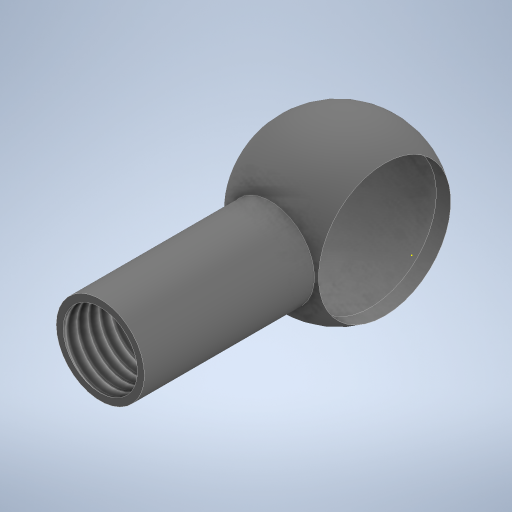
# Autodesk Inventor part: Part1
Saved by Autodesk Inventor 2023 (Build 270158000, 158)
## iProperties
Created: 2022-06-23
Part Number: Part1
Material: Stainless Steel
Document SubType Name: Modeling
Designer: earls
Density: 8 g/cm^3
Appearance: Gray
Author: earls
Autodesk Inventor part; units mm, degrees
ref_plane "YZ Plane" through (0, 0, 0) normal (1, 0, 0) x (0, 1, 0)
ref_plane "XZ Plane" through (0, 0, 0) normal (0, 1, 0) x (-1, 0, 0)
ref_plane "XY Plane" through (0, 0, 0) normal (0, 0, 1) x (1, 0, 0)
sketch "Sketch3" plane through (0, 0, 0) normal (1, 0, 0) x (0, 1, 0)
  line L0 (0, 0) -> (12, 0)
  circle A0 centre (0, 0) radius 11
  circle A1 centre (0, 0) radius 10
  line L1 (0, 0) -> (-14.3763, 0)
  point P0 (-11, 0)
  point P1 (-10, 0)
  point P2 (10, 0)
  point P3 (11, 0)
  dimension "d4" = 12
  dimension "d5" = 22
  dimension "d6" = 1
  constraints: 4 end point, 2 centre point, 2 horizontal, 1 coincident
  measures "d4" distance of L0.start L0.end
  measures "d5" diameter of A0
  measures "d6" radial gap between concentric circles of A0 A1
revolve "Revolution2" add sketch "Sketch3" angle 360 about axis through (0, 0, 0) along (0, 1, 0) picked at (-4.5651, 9.5627) contours A1 L1 A0 L0
sketch "Sketch4" plane through (0, 0, 0) normal (1, 0, 0) x (0, 1, 0)
  circle A0 centre (0, 0) radius 9
  circle A1 centre (0, 0) radius 10 projected
  dimension "d8" = 18
  constraints: 1 centre point, 1 coincident
  measures "d8" diameter of A0
extrude "Extrusion1" cut sketch "Sketch4" along normal blind 10 contours A0
sketch "Sketch5" plane through (10, 0, 0) normal (-1, 0, 0) x (0, 0, 1)
  point P0 (0, 0)
sketch "Sketch6" plane through (0, 0, 0) normal (1, 0, 0) x (0, 1, 0)
  circle A0 centre (0, 0) radius 4.5826 projected
extrude "Extrusion2" cut sketch "Sketch6" along normal blind 28.25
sketch "Sketch7" plane through (0, 0, 0) normal (0, 0, 1) x (1, 0, 0)
  circle A0 centre (0, 0) radius 6
  circle A1 centre (0, 0) radius 5.05
  dimension "d13" = 12
  dimension "d14" = 10.1
  constraints: 2 centre point, 2 coincident
  measures "d13" diameter of A0
  measures "d14" diameter of A1
extrude "Extrusion3" add sketch "Sketch7" along normal blind 32.34
sketch "Sketch8" plane through (0, 0, 0) normal (1, 0, 0) x (0, 1, 0)
  circle A0 centre (0, 0) radius 11
  line L0 (0, 0) -> (0, 12.838)
  line L1 (6, 0) -> (-6, 0) projected
  line L2 (0, 0) -> (0, -14.7719)
  circle A1 centre (0, 0) radius 10
  point P0 (0, 10)
  point P1 (0, -10)
  dimension "d17" = 1
  constraints: 4 end point, 2 centre point, 1 coincident, 1 perpendicular, 1 vertical
  measures "d17" radial gap between concentric circles of A0 A1
revolve "Revolution3" cut sketch "Sketch8" angle 360 about axis through (0, 0, 0) along (0, 0, -1) picked at (-0.7977, -6.5698) contours L0 L2 A1
thread "Thread1" size "M11x1.5" class "6H" standard "ANSI Metric M Profile" full length
sketch "Sketch10" plane through (0, 0, 0) normal (1, 0, 0) x (0, 1, 0)
  circle A0 centre (0, 0) radius 9
  dimension "d21" = 18
  constraints: 1 centre point, 1 coincident
  measures "d21" diameter of A0
extrude "Extrusion4" cut sketch "Sketch10" along normal blind 32.34
body "Solid2"
